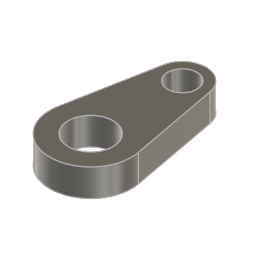
servo arm (Autodesk Fusion 360 design; units mm, degrees)
Autodesk Fusion 360 part; units mm, degrees
sketch "Sketch1" plane through (0, 0, 0) normal (0, 0, 1) x (1, 0, 0)
  circle A0 centre (0, 0) radius 2.45
  line L0 (0, 0) -> (0, 10) construction
  circle A1 centre (0, 10) radius 1.6
  circle A2 centre (0, 0) radius 4.45
  circle A3 centre (0, 10) radius 2.6
  line L1 (2.5551, 10.481) -> (4.3732, 0.8233)
  line L2 (-2.5551, 10.481) -> (-4.3732, 0.8232)
  dimension "d1" = 4.9
  dimension "d2" = 10
  dimension "d3" = 3.2
  dimension "d4" = 2
  dimension "d5" = 1
  constraint coincident A0.centre L0.start
  constraint vertical L0
  constraint coincident L0.end A1.centre
  constraint tangent A3 L1
  constraint tangent A2 L1
  constraint coincident A3 L1.start
  constraint coincident A2 L1.end
  constraint coincident A3 L2.start
  constraint tangent A3 L2
  constraint tangent A2 L2
  measures "d1" diameter of A0
  measures "d2" distance of A0.centre L0.end
  measures "d3" diameter of A1
extrude "Extrude1" add sketch "Sketch1" along normal blind 3
named bodies: "servo arm"
